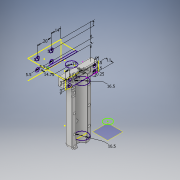
# Autodesk Inventor part: bottom_heating_lid
Saved by Autodesk Inventor 2018 (Build 220112000, 112)
## iProperties
Created: 2018-09-20
Part Number: bottom_heating_lid
Material: Generic
Document SubType Name: Modeling
Designer: Iek Man Lei
Density: 1 g/cm^3
Appearance: Default
Author: Iek Man Lei
Autodesk Inventor part; units mm, degrees
ref_plane "YZ Plane" through (0, 0, 0) normal (1, 0, 0) x (0, 1, 0)
ref_plane "XZ Plane" through (0, 0, 0) normal (0, 1, 0) x (-1, 0, 0)
ref_plane "XY Plane" through (0, 0, 0) normal (0, 0, 1) x (1, 0, 0)
sketch "Sketch1" plane through (0, 0, 0) normal (0, 1, 0) x (-1, 0, 0)
  line L0 (29.4, 24) -> (-24.6, 24)
  line L1 (-24.6, 24) -> (-24.6, -24)
  line L2 (-24.6, -24) -> (29.4, -24)
  line L3 (29.4, -24) -> (29.4, 24)
  line L4 (25.4, 20.15) -> (5.1, 20.15)
  line L5 (5.1, 20.15) -> (5.1, -20.15)
  line L6 (5.1, -20.15) -> (25.4, -20.15)
  line L7 (25.4, -20.15) -> (25.4, 20.15)
  point P0 (0, 0)
  dimension "d0" = 48
  dimension "d1" = 20.3
  dimension "d2" = 40.3
  dimension "d3" = 3.85
  dimension "d6" = 4
  dimension "d15" = 54
  constraints: 16 end point, 4 parallel, 2 horizontal, 2 perpendicular
  measures "d0" distance of L2.end L0.start
  measures "d1" distance of L6.end L5.end
  measures "d2" distance of L6.end L4.start
  measures "d3" distance between parallel lines of L2 L6
  measures "d6" distance between parallel lines of L3 L7
  measures "d15" distance of L1.end L2.end
extrude "Extrusion1" add sketch "Sketch1" along normal blind 13
sketch "Sketch2" plane through (0, 13, 0) normal (0, 1, 0) x (1, 0, 0)
  circle A0 centre (9.65, 0) radius 6.5
  line L0 (-29.4, -24) -> (24.6, -24) projected
  line L1 (-5.1, 20.15) -> (-5.1, -20.15) projected
  line L2 (-5.1, 20.15) -> (-25.4, 20.15) projected
  line L3 (-5.1, 20.15) -> (-2.1, 20.15)
  line L4 (-2.1, 20.15) -> (-2.1, -20.35)
  line L5 (-2.1, -20.35) -> (-5.1, -20.35)
  line L6 (-5.1, -20.35) -> (-5.1, 20.15)
  point P0 (0, 0)
  dimension "d7" = 13
  dimension "d8" = 24
  dimension "d14" = 14.75
  dimension "d28" = 3
  constraints: 8 end point, 2 parallel, 1 centre point, 1 horizontal, 1 perpendicular
  measures "d7" diameter of A0
  measures "d8" distance from line of L0 A0.centre
  measures "d14" distance from line of L1 A0.centre
  measures "d28" distance of L4.end L5.end
fillet "Fillet1" radius 2 2 edges at (24.6, 6.5, 24) (24.6, 6.5, -24)
fillet "Fillet4" radius 1 1 edges at (-5.1, 13, 0)
sketch "Sketch11" plane through (0, 0, 0) normal (0, -1, 0) x (1, 0, 0)
  line L0 (-29.4, 24) -> (22.6, 24) projected
  line L1 (-29.4, -24) -> (-0.9, -24)
  line L2 (-0.9, -24) -> (-0.9, 24)
  line L3 (-0.9, 24) -> (-29.4, 24)
  line L4 (-29.4, 24) -> (-29.4, -24)
  line L5 (-25.4, -20.15) -> (-4.1, -20.15) projected
  line L6 (-5.1, -20.15) -> (-5.1, 20.15) projected
  line L7 (-25.4, -20.15) -> (-5.1, -20.15)
  line L8 (-5.1, -20.15) -> (-5.1, 20.15)
  line L9 (-5.1, 20.15) -> (-25.4, 20.15)
  line L10 (-25.4, 20.15) -> (-25.4, -20.15)
  point P0 (0, 0)
  dimension "d92" = 28.5
  constraints: 16 end point, 4 parallel, 2 horizontal, 2 perpendicular, 1 point on line
  measures "d92" distance of L3.end L2.end
extrude "Extrusion15" add sketch "Sketch11" along normal blind 15
sketch "Sketch12" plane through (22.6, 13, -24) normal (0, 0, -1) x (-1, 0, 0)
  circle A0 centre (37.75, -5) radius 2.75
  circle A1 centre (38.1, -18) radius 2.75
  line L0 (48, -28) -> (48, 0) projected
  line L1 (0, 0) -> (52, 0) projected
  line L2 (52, -28) -> (23.5, -28) projected
  point P0 (22.6, -13)
  dimension "d96" = 5.5
  dimension "d97" = 5.5
  dimension "d100" = 10
  dimension "d125" = 5
  constraints: 2 centre point
  measures "d96" diameter of A0
  measures "d97" diameter of A1
  measures "d100" distance from line of L2 A1.centre
  measures "d125" distance from line of L1 A0.centre
extrude "Extrusion16" cut sketch "Sketch12" against normal through all
sketch "Sketch13" plane through (-29.4, 13, -24) normal (-1, 0, 0) x (0, 0, 1)
  circle A0 centre (14, -7) radius 2.75
  circle A1 centre (34, -7) radius 2.75
  circle A2 centre (34, -21) radius 2.75
  circle A3 centre (14, -21) radius 2.75
  line L0 (0, -28) -> (0, 0) projected
  line L1 (0, 0) -> (48, 0) projected
  line L2 (48, -28) -> (0, -28) projected
  point P0 (24, -13)
  dimension "d104" = 5.5
  dimension "d105" = 5.5
  dimension "d106" = 5.5
  dimension "d107" = 5.5
  dimension "d110" = 14
  dimension "d111" = 20
  dimension "d113" = 7
  dimension "d122" = 7
  constraints: 4 centre point, 2 horizontal alignment, 2 vertical alignment
  measures "d104" diameter of A0
  measures "d105" diameter of A1
  measures "d106" diameter of A2
  measures "d107" diameter of A3
  measures "d110" distance from line of L0 A0.centre
  measures "d111" distance of A0.centre A1.centre
  measures "d113" distance from line of L1 A0.centre
  measures "d122" distance from line of L2 A3.centre
extrude "Extrusion17" cut sketch "Sketch13" against normal blind 5.5
extrude "Extrusion19" cut sketch "Sketch13" against normal blind 40 contours A2 | A3
sketch "Sketch15" plane through (0, 13, 0) normal (0, 1, 0) x (1, 0, 0)
  line L0 (19.6, -13.25) -> (24.6, -13.25)
  line L1 (24.6, -13.25) -> (24.6, 12.75)
  line L2 (24.6, 12.75) -> (19.6, 12.75)
  line L3 (19.6, 12.75) -> (19.6, -13.25)
  line L4 (24.6, -22) -> (24.6, 22) projected
  line L5 (-27.4, 23.5) -> (22.6, 23.5) projected
  line L6 (22.6, 24) -> (-27.4, 24) projected
  line L7 (24.6, -13.25) -> (19.6, -13.25)
  line L8 (24.6, 12.75) -> (19.6, 12.75)
  line L9 (19.6, 0.75) -> (19.6, -1.25)
  line L10 (24.6, -22) -> (24.6, 22) projected
  circle A0 centre (24.6, 0) radius 8
  line L11 (19.6, 12.75) -> (16.15, 0)
  circle A1 centre (9.65, 0) radius 6.5 projected
  line L12 (16.15, 0) -> (19.6, -13.25)
  point P0 (0, 0)
  point P1 (24.6, 5)
  dimension "d149" = 5
  dimension "d150" = 0
  dimension "d151" = 26
  dimension "d154" = 11.25
  dimension "d155" = 5
  dimension "d156" = 12
  dimension "d157" = 12
  dimension "d158" = 5
  dimension "d234" = 16
  constraints: 18 end point, 5 point on line, 2 parallel, 1 centre point, 1 horizontal, 1 horizontal alignment, 1 midpoint, 1 perpendicular, 1 other
  measures "d149" distance of L2.end L1.end
  measures "d150" distance between parallel lines of L4 L1
  measures "d151" distance of L0.end L1.end
  measures "d154" distance between parallel lines of L6 L2
  measures "d155" distance of L0.end L7.end
  measures "d156" distance of L2.end L9.start
  measures "d157" distance of L0.start L9.end
  measures "d158" distance of L1.end L11.start
  measures "d234" diameter of A0
extrude "Extrusion22" cut sketch "Sketch15" against normal blind 8.5 contours L3 A0 L1 L0 | L12 L11 L3 A0 | A0 L3 | L3 A0 L1 | L3 L2 L1 A0
extrude "Extrusion23" add sketch "Sketch15" against normal blind 2.3 contours L3 A0 L1 L0 | L12 L11 L3 A0 | A0 L3 | L3 A0 L1 | L3 L2 L1 A0
sketch "Sketch16" plane through (0, 13, 0) normal (0, 1, 0) x (1, 0, 0)
  line L0 (23.1, -4.5) -> (24.6, -4.5)
  line L1 (24.6, -4.5) -> (24.6, 4.5)
  line L2 (24.6, 4.5) -> (23.1, 4.5)
  line L3 (23.1, 4.5) -> (23.1, -4.5)
  line L4 (22.6, 24) -> (-27.4, 24) projected
  line L5 (24.6, -12.75) -> (24.6, 12.75) projected
  line L6 (24.6, 1) -> (19.6, 1)
  line L7 (19.6, 1) -> (19.6, -1)
  line L8 (19.6, -1) -> (24.6, -1)
  line L9 (24.6, -1) -> (24.6, 1)
  point P0 (0, 0)
  dimension "d163" = 1.5
  dimension "d164" = 9
  dimension "d165" = 19.5
  dimension "d166" = 5
  dimension "d167" = 2
  dimension "d168" = 23
  constraints: 16 end point, 4 parallel, 2 horizontal, 2 perpendicular, 1 collinear, 1 point on line
  measures "d163" distance of L2.end L1.end
  measures "d164" distance of L0.end L1.end
  measures "d165" distance between parallel lines of L4 L2
  measures "d166" distance of L8.end L7.end
  measures "d167" distance of L6.start L8.end
  measures "d168" distance between parallel lines of L4 L6
extrude "Extrusion24" cut sketch "Sketch16" against normal blind 3
sketch "Sketch17" plane through (0, 0, 0) normal (0, -1, 0) x (1, 0, 0)
  line L0 (24.6, -13.75) -> (13.6, -13.75)
  line L1 (13.6, -13.75) -> (13.6, 13.75)
  line L2 (13.6, 13.75) -> (24.6, 13.75)
  line L3 (24.6, 13.75) -> (24.6, -13.75)
  line L4 (24.6, -22) -> (24.6, -7.25) projected
  line L5 (1.8697, -24) -> (22.6, -24) projected
  circle A0 centre (24.6, 0) radius 8.25
  point P0 (0, 0)
  dimension "d171" = 27.5
  dimension "d172" = 11
  dimension "d173" = 10.25
  dimension "d232" = 16.5
  constraints: 8 end point, 2 parallel, 1 centre point, 1 collinear, 1 horizontal, 1 midpoint, 1 perpendicular
  measures "d171" distance of L0.end L1.end
  measures "d172" distance of L0.start L0.end
  measures "d173" distance between parallel lines of L5 L0
  measures "d232" diameter of A0
sketch "Sketch18" plane through (0, 0, 0) normal (0, -1, 0) x (1, 0, 0)
  point P0 (0, 0)
extrude "Extrusion27" add sketch "Sketch17" along normal blind 68.5 contours L0 L1 L2 L3 A0 | A0 L3 picked at (23.9419, 3.0034)
sketch "Sketch19" plane through (0, -68.5, 0) normal (0, -1, 0) x (1, 0, 0)
  line L0 (24.6, 7.25) -> (24.6, -7.25) projected
  circle A0 centre (24.6, 0) radius 7.25
  point P0 (0, 0)
  constraints: 1 centre point, 1 midpoint
extrude "Extrusion28" cut sketch "Sketch19" against normal blind 68.5
sketch "Sketch21" plane through (24.6, 0, 22) normal (1, 0, 0) x (0, 0, -1)
  circle A0 centre (11.5, -35.5) radius 1.75
  circle A1 centre (11.5, -61.5) radius 1.75
  circle A2 centre (32.5, -9.5) radius 1.75
  circle A3 centre (32.5, -61.5) radius 1.75
  circle A4 centre (32.5, -35.5) radius 1.75
  line L0 (8.25, 0) -> (8.25, -68.5) projected
  line L1 (35.75, 0) -> (35.75, -68.5) projected
  circle A5 centre (11.5, -9.5) radius 1.75
  line L2 (14.75, -68.5) -> (8.25, -68.5) projected
  point P0 (22, 0)
  dimension "d183" = 3.5
  dimension "d184" = 3.5
  dimension "d185" = 3.5
  dimension "d186" = 3.5
  dimension "d198" = 3.5
  dimension "d199" = 3.25
  dimension "d200" = 3.25
  dimension "d201" = 3.5
  dimension "d202" = 7
  dimension "d203" = 26
  dimension "d204" = 26
  constraints: 6 centre point, 4 vertical alignment, 3 horizontal alignment
  measures "d183" diameter of A0
  measures "d184" diameter of A1
  measures "d185" diameter of A2
  measures "d186" diameter of A3
  measures "d198" diameter of A4
  measures "d199" distance from line of L0 A1.centre
  measures "d200" distance from line of L1 A3.centre
  measures "d201" diameter of A5
  measures "d202" distance from line of L2 A1.centre
  measures "d203" distance of A5.centre A0.centre
  measures "d204" distance of A1.centre A0.centre
sketch "Sketch22" plane through (0, -68.5, 0) normal (0, -1, 0) x (1, 0, 0)
  line L0 (24.6, 7.25) -> (24.6, -7.25) projected
  circle A0 centre (24.6, 0) radius 8.25
  point P0 (0, 0)
  dimension "d233" = 16.5
  constraints: 1 centre point, 1 midpoint
  measures "d233" diameter of A0
sketch "Sketch23" plane through (0, -68.5, 0) normal (0, -1, 0) x (1, 0, 0)
  circle A0 centre (25.4, -36.5125) radius 5.7238
  point P0 (0, 0)
  constraints: 1 centre point
ref_plane "Work Plane1" through (25.4, -81.5, -36.5125) normal (0, -1, 0) x (1, 0, 0)
sketch "Sketch24" plane through (25.4, -81.5, -36.5125) normal (0, -1, 0) x (1, 0, 0)
  line L0 (-0.8, 43.7625) -> (-0.8, 29.2625) projected
  circle A0 centre (-0.8, 36.5125) radius 5.75
  point P0 (-25.4, 36.5125)
  dimension "d189" = 11.5
  constraints: 1 centre point, 1 midpoint
  measures "d189" diameter of A0
extrude "Extrusion30" add sketch "Sketch17" along normal blind 81.5 contours L0 L1 L2 L3 A0 | A0 L3 picked at (23.9419, 3.0034)
extrude "Extrusion31" cut sketch "Sketch22" against normal blind 76
loft "Loft1" cut profiles "Sketch22", "Sketch24"
sketch "Sketch25" plane through (24.6, 0, 22) normal (1, 0, 0) x (0, 0, -1)
  circle A0 centre (4, 10) radius 2.25
  circle A1 centre (4, 3) radius 2.25
  circle A2 centre (40, 10) radius 2.25
  circle A3 centre (40, 3) radius 2.25
  line L0 (-2, 13) -> (-2, 0) projected
  line L1 (46, 0) -> (46, 13) projected
  line L2 (0, 13) -> (17.5, 13) projected
  line L3 (0, 0) -> (8.25, 0) projected
  point P0 (22, 0)
  dimension "d205" = 4.5
  dimension "d206" = 4.5
  dimension "d207" = 4.5
  dimension "d208" = 4.5
  dimension "d209" = 6
  dimension "d210" = 6
  dimension "d211" = 3
  dimension "d212" = 3
  constraints: 4 centre point, 2 horizontal alignment, 2 vertical alignment
  measures "d205" diameter of A0
  measures "d206" diameter of A1
  measures "d207" diameter of A2
  measures "d208" diameter of A3
  measures "d209" distance from line of L0 A0.centre
  measures "d210" distance from line of L1 A2.centre
  measures "d211" distance from line of L2 A0.centre
  measures "d212" distance from line of L3 A1.centre
extrude "Extrusion32" cut sketch "Sketch25" against normal blind 3.5
extrude "Extrusion34" cut sketch "Sketch21" against normal blind 2.5
sketch "Sketch26" plane through (24.6, 0, 22) normal (1, 0, 0) x (0, 0, -1)
  circle A0 centre (32.25, -76.5) radius 1.65
  circle A1 centre (11.75, -76.5) radius 1.65
  line L0 (8.25, 0) -> (8.25, -81.5) projected
  line L1 (35.75, 0) -> (35.75, -81.5) projected
  line L2 (35.75, -81.5) -> (8.25, -81.5) projected
  point P0 (22, 0)
  point P1 (16.25, -81.5)
  dimension "d219" = 3.3
  dimension "d220" = 3.3
  dimension "d221" = 3.5
  dimension "d222" = 3.5
  dimension "d223" = 5
  constraints: 2 centre point, 1 horizontal alignment
  measures "d219" diameter of A0
  measures "d220" diameter of A1
  measures "d221" distance from line of L0 A1.centre
  measures "d222" distance from line of A0.centre L1
  measures "d223" distance from line of L2 A1.centre
extrude "Extrusion35" cut sketch "Sketch26" against normal blind 2.3
fillet "Fillet14" radius 3 2 edges at (19.1, 0, 13.75) (19.1, 0, -13.75)
fillet "Fillet15" radius 5 2 edges at (19.1, -81.5, 13.75) (19.1, -81.5, -13.75)
fillet "Fillet16" radius 3 7 edges at (13.6, -80.0355, -12.2855) (13.6, -39.75, -13.75) (13.6, -0.8787, -14.6287) (13.6, -80.0355, 12.2855) (13.6, -39.75, 13.75) (13.6, -0.8787, 14.6287) (13.6, -81.5, 0)
fillet "Fillet17" radius 1 26 edges at (24.6, -80.0355, -12.2855) (24.6, -81.5, -7.25) (24.6, -0.8787, -14.6287) (24.6, 0, -19.375) (24.0142, 0, -23.4142) (10.85, 0, -24) (24.6, -39.75, -13.75) (24.6, -80.0355, 12.2855) (24.6, -81.5, 7.25) (24.6, -0.8787, 14.6287) (24.6, 0, 19.375) (24.0142, 0, 23.4142) (10.85, 0, 24) (24.6, -39.75, 13.75) (24.0142, 13, -23.4142) (24.6, 13, -13.25) (-3.4, 13, -24) (24.0142, 13, 23.4142) (24.6, 13, 13.25) (-3.4, 13, 24) (-14.75, 13, 20.15) (-14.75, 13, -20.15) (-15.25, -15, -20.15) (-5.1, -15, 0) (-25.4, -15, 0) (-15.25, -15, 20.15)
fillet "Fillet18" radius 0.5 35 edges at (24.6, -32, 8.25) (24.3411, -81.1714, 5.8074) (18.85, -81.5, 0) (24.3411, -81.1714, -5.8074) (24.6, -74.5, -7.0962) (24.6, -74.5, 7.0962) (24.6, -32, -8.25) (20.0927, 4.5, -6.9099) (16.3501, 4.5, 0.0339) (19.9988, 4.5, 6.8478) (19.6, 10.7, 0) (21.35, 10.7, -1) (21.35, 10.7, 1) (23.1, 10.7, 2.75) (23.1, 13, 2.75) (23.1, 11.85, -1) (21.35, 13, -1) (23.1, 10.7, -2.75) (23.1, 13, -2.75) (24.3071, 12.7071, -4.5) (23.35, 13, -4.5) (24.6, 11.35, -4.5) (23.85, 10.7, -4.5) (24.6, 10.7, -8.625) (24.6, 7.6, -12.75) (24.6, 4.5, -10.5) (24.6, 10.7, 8.875) (24.6, 4.5, 10.75) (19.6, 7.6, -12.75) (24.3071, 12.7071, 4.5) (23.35, 13, 4.5) (24.6, 11.35, 4.5) (23.1, 11.85, 1) (21.35, 13, 1) (19.6, 13, 0)
sketch "Sketch28" plane through (16.6, -76.5, -13.75) normal (0, 0, -1) x (-1, 0, 0)
  point P0 (16.6, 76.5)
sketch "Sketch29" plane through (0, 0, 0) normal (0, 0, 1) x (1, 0, 0)
  circle A0 centre (24.1, -3) radius 1
  circle A1 centre (24.1, -6) radius 1
  line L0 (23.6, -3) -> (16.6, -3) projected
  line L1 (24.6, -3) -> (24.6, -76.5) projected
  line L2 (43.2297, -81.5) -> (-41.5115, -81.5) projected
  circle A2 centre (24.1, -13.5) radius 1
  point P0 (0, 0)
  dimension "d235" = 2
  dimension "d236" = 2
  dimension "d237" = 3
  dimension "d238" = 0
  dimension "d241" = 0.5
  dimension "d262" = 2
  dimension "d263" = 0.5
  dimension "d264" = 0.5
  dimension "d265" = 68
  constraints: 3 centre point
  measures "d235" diameter of A0
  measures "d236" diameter of A1
  measures "d237" distance of A1.centre A0.centre
  measures "d238" distance from line of L0 A0.centre
  measures "d241" distance from line of L1 A0.centre
  measures "d262" diameter of A2
  measures "d263" distance from line of A2.centre L1
  measures "d264" distance from line of L1 A1.centre
  measures "d265" distance from line of L2 A2.centre
extrude "Extrusion36" cut sketch "Sketch29" along normal through all
sketch "Sketch30" plane through (0, 0, 0) normal (0, -1, 0) x (1, 0, 0)
  line L0 (-39.6875, 36.5125) -> (13.6, 36.5125)
  line L1 (13.6, -34.925) -> (-39.6875, -34.925)
  line L2 (-39.6875, -34.925) -> (-39.6875, 36.5125)
  line L3 (24.6, 19.0308) -> (24.6, 22) projected
  line L4 (13.6, -34.925) -> (13.6, 36.5125)
  line L5 (13.6, 8.75) -> (13.6, -8.75) projected
  point P0 (0, 0)
  dimension "d260" = 71.4375
  constraints: 8 end point, 1 collinear, 1 horizontal, 1 parallel, 1 vertical
  measures "d260" distance of L0.end L1.start
extrude "Extrusion37" cut sketch "Sketch30" along normal mid plane 30
sketch "Sketch31" plane through (13.6, -76.5, -10.75) normal (-1, 0, 0) x (0, 0, 1)
  circle A0 centre (10.75, 22) radius 2.5
  line L0 (2, -5) -> (19.5, -5) projected
  line L1 (24.5, 0) -> (24.5, 73.5) projected
  point P0 (10.75, 76.5)
  dimension "d247" = 5
  dimension "d248" = 27
  dimension "d249" = 13.75
  constraints: 1 centre point
  measures "d247" diameter of A0
  measures "d248" distance from line of A0.centre L0
  measures "d249" distance from line of A0.centre L1
extrude "Extrusion38" cut sketch "Sketch31" against normal blind 10
sketch "Sketch32" plane through (22.6, 1, 24) normal (0, 0, 1) x (1, 0, 0)
  circle A0 centre (1, 5.5) radius 1.25
  line L0 (0, 12) -> (-9, 12) projected
  line L1 (2, 0) -> (2, 11) projected
  point P0 (-22.6, -1)
  point P1 (-10, 12)
  dimension "d252" = 2.5
  dimension "d253" = 6.5
  dimension "d254" = 1
  constraints: 1 centre point
  measures "d252" diameter of A0
  measures "d253" distance from line of A0.centre L0
  measures "d254" distance from line of A0.centre L1
extrude "Extrusion39" cut sketch "Sketch32" against normal blind 13
sketch "Sketch33" plane through (0, 13, 0) normal (0, 1, 0) x (1, 0, 0)
  line L0 (23.1, -8.1125) -> (23.1, -13.75) projected
  circle A0 centre (23.1, -9.525) radius 1.25
  point P0 (0, 0)
  dimension "d257" = 2.5
  constraints: 1 centre point, 1 point on line
  measures "d257" diameter of A0
extrude "Extrusion40" cut sketch "Sketch33" against normal blind 5
fillet "Fillet19" radius 2 9 edges at (13.6, 0.2929, 23.7071) (13.6, 6.5, 24) (13.6, 12.7071, 23.7071) (13.6, 13, 0) (13.6, 12.7071, -23.7071) (13.6, 6.5, -24) (13.6, 0.2929, -23.7071) (13.6, 0, -17.2769) (13.6, 0, 17.2769)
equation "\"d115\" = d107"
body "Solid1"
